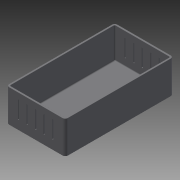
# Autodesk Inventor part: Box_Square_Bottom
Saved by Autodesk Inventor 2015 (Build 190159000, 159)
## iProperties
Created: 2014-09-24
Part Number: Box_Square_Bottom
Material: Generic
Document SubType Name: Modeling
Designer: Jake
Density: 1 g/cm^3
Appearance: Light Gray
Author: Jake
Autodesk Inventor part; units mm, degrees
ref_plane "YZ Plane" through (0, 0, 0) normal (1, 0, 0) x (0, 1, 0)
ref_plane "XZ Plane" through (0, 0, 0) normal (0, 1, 0) x (-1, 0, 0)
ref_plane "XY Plane" through (0, 0, 0) normal (0, 0, 1) x (1, 0, 0)
sketch "Sketch1" plane through (0, 0, 0) normal (0, 1, 0) x (-1, 0, 0)
  line L0 (63.5, 34.5) -> (-63.5, 34.5)
  line L1 (-63.5, 34.5) -> (-63.5, -34.5)
  line L2 (-63.5, -34.5) -> (63.5, -34.5)
  line L3 (63.5, -34.5) -> (63.5, 34.5)
  line L4 (63.5, 34.5) -> (-63.5, -34.5) construction
  line L5 (-63.5, 34.5) -> (63.5, -34.5) construction
  point P0 (0, 0)
  dimension "d0" = 127
  dimension "d1" = 69
  constraints: 12 end point, 2 midpoint, 2 parallel, 1 horizontal, 1 perpendicular
  measures "d0" distance of L2.end L1.end
  measures "d1" distance of L1.end L0.end
extrude "Extrusion1" add sketch "Sketch1" along normal blind 38.1
fillet "Fillet1" radius 3.175 8 edges at (63.5, 19.05, 34.5) (63.5, 19.05, -34.5) (-63.5, 19.05, -34.5) (-63.5, 19.05, 34.5) (0, 0, 34.5) (63.5, 0, 0) (0, 0, -34.5) (-63.5, 0, 0)
shell "Shell1" thickness 2 removed faces 1 at (20.1083, 38.1, -11.5)
sketch "Sketch2" plane through (-63.5, 3.175, 31.325) normal (-1, 0, 0) x (0, 0, 1)
  line L0 (-31.615, 7.4625) -> (-30.615, 7.4625)
  line L1 (-30.615, 7.4625) -> (-30.615, 27.4625)
  line L2 (-30.615, 27.4625) -> (-31.615, 27.4625)
  line L3 (-31.615, 27.4625) -> (-31.615, 7.4625)
  line L4 (-31.615, 7.4625) -> (-30.615, 27.4625) construction
  line L5 (-30.615, 7.4625) -> (-31.615, 27.4625) construction
  point P0 (-31.325, -3.175)
  point P1 (-31.115, 17.4625)
  dimension "d6" = 1
  dimension "d7" = 20
  constraints: 12 end point, 2 midpoint, 2 parallel, 1 horizontal, 1 perpendicular
  measures "d6" distance of L2.end L1.end
  measures "d7" distance of L1.end L0.end
extrude "Extrusion2" cut sketch "Sketch2" against normal blind 10
pattern_linear "Rectangular Pattern1" count 5 spacing 10 along (0, 0, 1) of "Extrusion2" first direction both ways yes
mirror "Mirror1" about plane through (0, 0, 0) normal (1, 0, 0) of "Extrusion2", "Rectangular Pattern1"
fillet "Fillet2" radius 0.25 40 edges at (-62.5, 30.6375, -20.29) (-62.5, 30.6375, -19.29) (-62.5, 10.6375, -19.29) (-62.5, 10.6375, -20.29) (-62.5, 30.6375, -10.29) (-62.5, 30.6375, -9.29) (-62.5, 10.6375, -9.29) (-62.5, 10.6375, -10.29) (-62.5, 30.6375, -0.29) (-62.5, 30.6375, 0.71) (-62.5, 10.6375, 0.71) (-62.5, 10.6375, -0.29) (-62.5, 30.6375, 9.71) (-62.5, 30.6375, 10.71) (-62.5, 10.6375, 10.71) (-62.5, 10.6375, 9.71) (-62.5, 30.6375, 19.71) (-62.5, 30.6375, 20.71) (-62.5, 10.6375, 20.71) (-62.5, 10.6375, 19.71) (62.5, 10.6375, 19.71) (62.5, 30.6375, 19.71) (62.5, 10.6375, 20.71) (62.5, 30.6375, 20.71) (62.5, 10.6375, 9.71) (62.5, 30.6375, 9.71) (62.5, 10.6375, 10.71) (62.5, 30.6375, 10.71) (62.5, 10.6375, -0.29) (62.5, 30.6375, -0.29) (62.5, 30.6375, 0.71) (62.5, 10.6375, 0.71) (62.5, 10.6375, -10.29) (62.5, 30.6375, -10.29) (62.5, 10.6375, -9.29) (62.5, 30.6375, -9.29) (62.5, 10.6375, -20.29) (62.5, 30.6375, -20.29) (62.5, 10.6375, -19.29) (62.5, 30.6375, -19.29)
fillet "Fillet3" radius 0.25 176 edges at (-63.5, 30.6375, -19.79) (-63.5, 30.5643, -19.3632) (-63.5, 30.5643, -20.2168) (-63.5, 20.6375, -19.29) (-63.5, 20.6375, -20.29) (-63.5, 10.7107, -19.3632) (-63.5, 10.7107, -20.2168) (-63.5, 10.6375, -19.79) (-63.5, 38.1, 0) (-63.5, 30.6375, -9.79) (-63.5, 30.5643, -9.3632) (-63.5, 30.5643, -10.2168) (-63.5, 20.6375, -9.29) (-63.5, 20.6375, -10.29) (-63.5, 10.7107, -9.3632) (-63.5, 10.7107, -10.2168) (-63.5, 10.6375, -9.79) (-63.5, 30.6375, 0.21) (-63.5, 30.5643, 0.6368) (-63.5, 30.5643, -0.2168) (-63.5, 20.6375, 0.71) (-63.5, 20.6375, -0.29) (-63.5, 10.7107, 0.6368) (-63.5, 10.7107, -0.2168) (-63.5, 10.6375, 0.21) (-63.5, 30.6375, 10.21) (-63.5, 30.5643, 10.6368) (-63.5, 30.5643, 9.7832) (-63.5, 20.6375, 10.71) (-63.5, 20.6375, 9.71) (-63.5, 10.7107, 10.6368) (-63.5, 10.7107, 9.7832) (-63.5, 10.6375, 10.21) (-63.5, 30.6375, 20.21) (-63.5, 30.5643, 20.6368) (-63.5, 30.5643, 19.7832) (-63.5, 20.6375, 20.71) (-63.5, 20.6375, 19.71) (-63.5, 10.7107, 20.6368) (-63.5, 10.7107, 19.7832) (-63.5, 10.6375, 20.21) (-61.5, 30.6375, -19.79) (-61.5, 30.5643, -19.3632) (-61.5, 30.5643, -20.2168) (-61.5, 20.6375, -19.29) (-61.5, 20.6375, -20.29) (-61.5, 10.7107, -19.3632) (-61.5, 10.7107, -20.2168) (-61.5, 10.6375, -19.79) (-62.5701, 38.1, 33.5701) (0, 38.1, 34.5) (62.5701, 38.1, 33.5701) (63.5, 38.1, 0) (62.5701, 38.1, -33.5701) (0, 38.1, -34.5) (-62.5701, 38.1, -33.5701) (-61.5, 38.1, 0) (-61.1559, 38.1, -32.1559) (0, 38.1, -32.5) (61.1559, 38.1, -32.1559) (61.5, 38.1, 0) (61.1559, 38.1, 32.1559) (0, 38.1, 32.5) (-61.1559, 38.1, 32.1559) (-61.5, 30.6375, -9.79) (-61.5, 30.5643, -9.3632) (-61.5, 30.5643, -10.2168) (-61.5, 20.6375, -9.29) (-61.5, 20.6375, -10.29) (-61.5, 10.7107, -9.3632) (-61.5, 10.7107, -10.2168) (-61.5, 10.6375, -9.79) (-61.5, 30.6375, 0.21) (-61.5, 30.5643, 0.6368) (-61.5, 30.5643, -0.2168) (-61.5, 20.6375, 0.71) (-61.5, 20.6375, -0.29) (-61.5, 10.7107, 0.6368) (-61.5, 10.7107, -0.2168) (-61.5, 10.6375, 0.21) (-61.5, 30.6375, 10.21) (-61.5, 30.5643, 10.6368) (-61.5, 30.5643, 9.7832) (-61.5, 20.6375, 10.71) (-61.5, 20.6375, 9.71) (-61.5, 10.7107, 10.6368) (-61.5, 10.7107, 9.7832) (-61.5, 10.6375, 10.21) (-61.5, 30.6375, 20.21) (-61.5, 30.5643, 20.6368) (-61.5, 30.5643, 19.7832) (-61.5, 20.6375, 20.71) (-61.5, 20.6375, 19.71) (-61.5, 10.7107, 20.6368) (-61.5, 10.7107, 19.7832) (-61.5, 10.6375, 20.21) (63.5, 20.6375, 19.71) (63.5, 30.5643, 19.7832) (63.5, 10.7107, 19.7832) (63.5, 30.6375, 20.21) (63.5, 10.6375, 20.21) (63.5, 30.5643, 20.6368) (63.5, 10.7107, 20.6368) (63.5, 20.6375, 20.71) (63.5, 20.6375, 9.71) (63.5, 30.5643, 9.7832) (63.5, 10.7107, 9.7832) (63.5, 30.6375, 10.21) (63.5, 10.6375, 10.21) (63.5, 30.5643, 10.6368) (63.5, 10.7107, 10.6368) (63.5, 20.6375, 10.71) (63.5, 20.6375, -0.29) (63.5, 30.5643, -0.2168) (63.5, 10.7107, -0.2168) (63.5, 30.6375, 0.21) (63.5, 10.6375, 0.21) (63.5, 30.5643, 0.6368) (63.5, 10.7107, 0.6368) (63.5, 20.6375, 0.71) (63.5, 20.6375, -10.29) (63.5, 30.5643, -10.2168) (63.5, 10.7107, -10.2168) (63.5, 30.6375, -9.79) (63.5, 10.6375, -9.79) (63.5, 30.5643, -9.3632) (63.5, 10.7107, -9.3632) (63.5, 20.6375, -9.29) (63.5, 20.6375, -20.29) (63.5, 30.5643, -20.2168) (63.5, 10.7107, -20.2168) (63.5, 30.6375, -19.79) (63.5, 10.6375, -19.79) (63.5, 30.5643, -19.3632) (63.5, 10.7107, -19.3632) (63.5, 20.6375, -19.29) (61.5, 10.6375, 20.21) (61.5, 10.7107, 20.6368) (61.5, 10.7107, 19.7832) (61.5, 20.6375, 20.71) (61.5, 20.6375, 19.71) (61.5, 30.5643, 20.6368) (61.5, 30.5643, 19.7832) (61.5, 30.6375, 20.21) (61.5, 10.6375, 10.21) (61.5, 10.7107, 10.6368) (61.5, 10.7107, 9.7832) (61.5, 20.6375, 10.71) (61.5, 20.6375, 9.71) (61.5, 30.5643, 10.6368) (61.5, 30.5643, 9.7832) (61.5, 30.6375, 10.21) (61.5, 10.6375, 0.21) (61.5, 10.7107, 0.6368) (61.5, 10.7107, -0.2168) (61.5, 20.6375, 0.71) (61.5, 20.6375, -0.29) (61.5, 30.5643, 0.6368) (61.5, 30.5643, -0.2168) (61.5, 30.6375, 0.21) (61.5, 10.6375, -9.79) (61.5, 10.7107, -9.3632) (61.5, 10.7107, -10.2168) (61.5, 20.6375, -9.29) (61.5, 20.6375, -10.29) (61.5, 30.5643, -9.3632) (61.5, 30.5643, -10.2168) (61.5, 30.6375, -9.79) (61.5, 10.6375, -19.79) (61.5, 10.7107, -19.3632) (61.5, 10.7107, -20.2168) (61.5, 20.6375, -19.29) (61.5, 20.6375, -20.29) (61.5, 30.5643, -19.3632) (61.5, 30.5643, -20.2168) (61.5, 30.6375, -19.79)
delete faces "Delete Face1" heal yes whole lump no faces at (-60.7982, 0.0355, -10.4417) (-61.7142, 2.5149, 34.1026) (-20.1083, 1.0155, 33.6524) (-20.1083, 0.0089, -31.5623) (-63.1026, 2.5149, -32.7142) (63.1026, 2.5149, -32.7142) (61.485, 0.2195, 10.4417) (61.7142, 2.5149, 34.1026)
move or copy body "Move Body1" bodies to move or copy 1 copy no rotation origin (0, 0, 0) rotation axis (1, 0, 0) rotation angle 90
body "Solid1"
